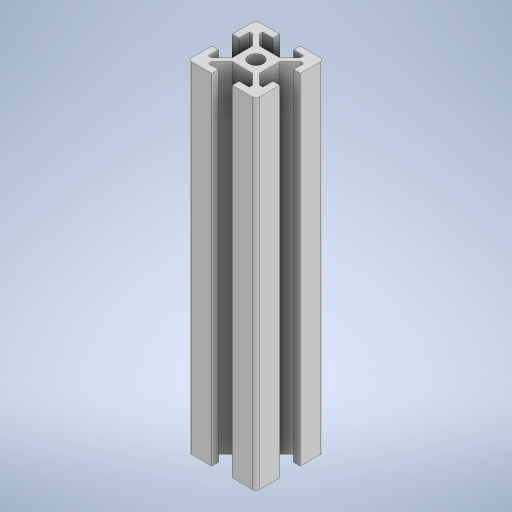
# Autodesk Inventor part: Балка 100 мм
Saved by Autodesk Inventor 2023 (Build 270158000, 158)
## iProperties
Created: 2022-04-25
Part Number: Балка 100 мм
Material: Типовые
Document SubType Name: Modeling
Designer: avkap
Density: 1 g/cm^3
Appearance: По умолчанию
Author: avkap
Autodesk Inventor part; units mm, degrees
ref_plane "YZ Plane" through (0, 0, 0) normal (1, 0, 0) x (0, 1, 0)
ref_plane "XZ Plane" through (0, 0, 0) normal (0, 1, 0) x (-1, 0, 0)
ref_plane "XY Plane" through (0, 0, 0) normal (0, 0, 1) x (1, 0, 0)
sketch "Эскиз1" plane through (0, 0, 0) normal (0, 1, 0) x (-1, 0, 0)
  circle A0 centre (0, 0) radius 2.1
  line L0 (0, 0) -> (3.9981, 0)
  line L1 (3.9981, 0) -> (3.9981, 3)
  line L2 (2.9981, 4) -> (-3.0019, 4)
  line L3 (-4.0019, 3) -> (-4.0019, -3)
  line L4 (-3, -4) -> (3, -4)
  line L5 (3.9981, -3) -> (3.9981, 3)
  line L6 (9.9956, 3.999) -> (9.9981, 8.999)
  line L7 (8.9983, 9.999) -> (7.9983, 9.999)
  line L8 (9.9976, 7.999) -> (9.9981, 8.999)
  line L9 (-10.0019, -3) -> (-10.0019, -6.0019)
  line L10 (9.9981, -9.0019) -> (9.9981, -2.9876)
  line L11 (9.9981, 3) -> (9.9981, 8.999)
  line L12 (7.9793, -5.9876) -> (7.9793, -2.9876)
  line L13 (7.9981, 3) -> (7.9981, 6)
  line L14 (6, -7) -> (6, -8)
  line L15 (-8, 5.9981) -> (-8, 3)
  line L16 (-8.0019, -3) -> (-8.0019, -6.0019)
  line L17 (-10.0019, -3) -> (-10.0019, -9.0019)
  line L18 (8.9983, 9.999) -> (2.9983, 9.999)
  line L19 (5.9981, 7.999) -> (2.9983, 7.999)
  line L20 (-3.0026, 8) -> (-6.0019, 8)
  line L21 (-8, 5.9981) -> (-7, 5.9981)
  line L22 (6.9981, 6) -> (7.9981, 6)
  line L23 (-8.0019, -6.0019) -> (-7.0024, -6.0019)
  line L24 (2.9981, -8) -> (6, -8)
  line L25 (-9.0019, -10.0019) -> (-3.0019, -10.0019)
  line L26 (2.9981, -10.0019) -> (8.9981, -10.0019)
  line L27 (8.9983, 9.999) -> (6.9981, 9.999)
  line L28 (9.9981, 6.999) -> (9.9981, 8.999)
  line L29 (8.9981, -10.0019) -> (6.9981, -10.0019)
  line L30 (9.9981, -7.0019) -> (9.9981, -9.0019)
  line L31 (-9.0019, -10.0019) -> (-7.0019, -10.0019)
  line L32 (-10.0019, -7.0019) -> (-10.0019, -9.0019)
  line L33 (5.9981, 7) -> (2.9981, 4)
  line L34 (6.9981, 6) -> (3.9981, 3)
  line L35 (-3.0019, 4) -> (-6.0019, 7)
  line L36 (-4.0019, 3) -> (-7, 5.9981)
  line L37 (-4.0019, -3) -> (-7.0024, -6.0019)
  line L38 (-6, -7) -> (-3, -4)
  line L39 (3, -4) -> (6, -7)
  line L40 (6.9857, -5.9876) -> (3.9981, -3)
  line L41 (6.9981, 9.999) -> (6.9981, 9.9981)
  line L42 (6.9981, 8.0054) -> (6.9981, 8)
  line L43 (2.9983, 9.999) -> (2.9983, 7.999)
  line L44 (7.9981, 3) -> (9.9981, 3)
  line L45 (9.9981, -2.9876) -> (7.9793, -2.9876)
  line L46 (6.9857, -5.9876) -> (7.9793, -5.9876)
  line L47 (2.9981, -8) -> (2.9981, -10.0019)
  line L48 (-6, -7) -> (-6, -8)
  line L49 (-3.0019, -10.0019) -> (-3.0019, -8)
  line L50 (-2.9895, -5.9896) -> (-2.9895, -5.9876)
  line L51 (-3.0026, 8) -> (-3.0019, 9.9961)
  line L52 (-10, 3) -> (-8, 3)
  line L53 (-6, -8) -> (-3.0019, -8)
  line L54 (-6.0019, -5) -> (-6.0019, -5.001)
  line L55 (-8.0019, -3) -> (-10.0019, -3)
  line L56 (5.9981, 7.999) -> (5.9981, 7)
  line L57 (-6.0019, 8) -> (-6.0019, 7)
  line L58 (9.9981, 8.999) -> (9.9971, 8.999)
  line L59 (-10, 9) -> (-10, 8.9981)
  line L60 (-10.0019, -9.0029) -> (-10.0019, -9.0019)
  line L61 (-10.0019, -9.0019) -> (-10, -9.0019)
  line L62 (9.9981, -9.0019) -> (9.9805, -9.0019)
  arc A1 (9.9981, 8.999) -> (8.9983, 9.999) centre (8.9981, 8.999) ccw
  arc A2 (-10.0019, -9.0019) -> (-9.0019, -10.0019) centre (-9.0019, -9.0019) ccw
  arc A3 (8.9981, -10.0019) -> (9.9981, -9.0019) centre (8.9981, -9.0019) ccw
  line L63 (10, 10) -> (10, 9.999)
  line L64 (9.9981, 9.0175) -> (9.9981, 8.999)
  arc A4 (-8.998, 9.9961) -> (-10, 8.9981) centre (-9.0019, 8.9981) ccw
  line L65 (-10, 9) -> (-10, 8.9981)
  line L66 (-10, 3) -> (-10, 9)
  line L67 (-8.998, 9.9961) -> (-3.0019, 9.9961)
  point P0 (-10, 8.999)
  constraints: 136 end point, 32 perpendicular, 17 parallel, 13 point on line, 10 horizontal, 9 point on circle, 5 centre point, 1 coincident, 1 collinear, 1 midpoint, 1 vertical
extrude "Выдавливание1" add sketch "Эскиз1" along normal blind 100
